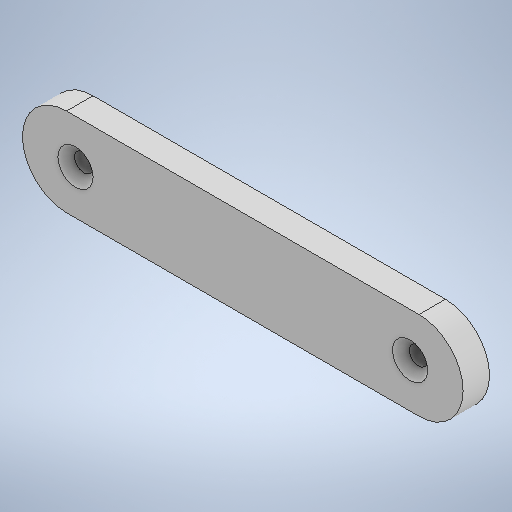
# Autodesk Inventor part: support_gopro
Saved by Autodesk Inventor 2025.2 (Build 292293000, 293)
## iProperties
Created: 2025-05-12
Part Number: support_gopro
Material: Générique
Document SubType Name: Modeling
Designer: enezl
Density: 1 g/cm^3
Appearance: Par défaut
Author: enezl
Autodesk Inventor part; units mm, degrees
ref_plane "YZ Plane" through (0, 0, 0) normal (1, 0, 0) x (0, 1, 0)
ref_plane "XZ Plane" through (0, 0, 0) normal (0, 1, 0) x (-1, 0, 0)
ref_plane "XY Plane" through (0, 0, 0) normal (0, 0, 1) x (1, 0, 0)
sketch "Esquisse1" plane through (0, 0, 0) normal (0, 0, 1) x (1, 0, 0)
  line L0 (-40, 0) -> (40, 0) construction
  line L1 (-40, -10) -> (40, -10)
  line L2 (40, 10) -> (-40, 10)
  arc A0 (-40, 10) -> (-40, -10) centre (-40, 0) ccw
  arc A1 (40, -10) -> (40, 10) centre (40, 0) ccw
  point P0 (0, 0)
  point P1 (0, 0)
  dimension "d0" = 20
  dimension "d1" = 80
  constraints: 8 end point, 4 point on circle, 4 tangent, 3 coincident, 2 centre point, 1 horizontal, 1 midpoint, 1 parallel
  measures "d0" distance between parallel lines of L1 L2
  measures "d1" distance of L0.start L0.end
extrude "Extrusion1" add sketch "Esquisse1" along normal blind 6
sketch "Esquisse2" plane through (0, 0, 6) normal (0, 0, 1) x (1, 0, 0)
  line L0 (-37.9704, 0) -> (37.9704, 0) construction
  point P0 (0, 0)
  point P1 (0, 0)
  constraints: 2 end point, 1 coincident, 1 horizontal, 1 midpoint
hole "Perçage1" at (-37.9704, 0, 6) at (37.9704, 0, 6) direction (0, 0, -1) diameter 4.2 depth 6 tip angle 118 start extended yes countersink diameter 8 countersink angle 90
